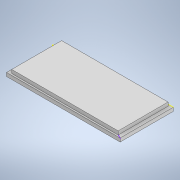
# Autodesk Inventor part: kansi
Saved by Autodesk Inventor 2020.1 (Build 241239000, 239)
## iProperties
Created: 2021-11-03
Part Number: kansi
Material: Generic
Document SubType Name: Modeling
Designer: s1mate03
Density: 1 g/cm^3
Appearance: Default
Author: s1mate03
Autodesk Inventor part; units mm, degrees
ref_plane "YZ Plane" through (0, 0, 0) normal (1, 0, 0) x (0, 1, 0)
ref_plane "XZ Plane" through (0, 0, 0) normal (0, 1, 0) x (-1, 0, 0)
ref_plane "XY Plane" through (0, 0, 0) normal (0, 0, 1) x (1, 0, 0)
sketch "Sketch1" plane through (0, 0, 0) normal (0, 1, 0) x (-1, 0, 0)
  line L0 (0, 13.1214) -> (-32, 13.1214)
  line L1 (-32, 13.1214) -> (-32, -1.8786)
  line L2 (-32, -1.8786) -> (0, -1.8786)
  line L3 (0, -1.8786) -> (0, 13.1214)
  point P0 (0, 0)
  dimension "d0" = 32
  dimension "d1" = 15
  constraints: 8 end point, 2 parallel, 1 horizontal, 1 perpendicular
  measures "d0" distance of L2.end L1.end
  measures "d1" distance of L1.end L0.end
extrude "Extrusion1" add sketch "Sketch1" along normal blind 1
sketch "Sketch2" plane through (0, 1, 0) normal (0, 1, 0) x (1, 0, 0)
  line L0 (32, 1.8786) -> (0, 1.8786) projected
  line L1 (32.1041, -13.1869) -> (0, 1.8786)
  point P0 (0, 0)
  constraints: 2 end point
sketch "Sketch3" plane through (0, 1, 0) normal (0, 1, 0) x (1, 0, 0)
  line L0 (31.001, -12.6665) -> (0.9997, -12.6665)
  line L1 (0.9997, -12.6665) -> (0.9997, 1.4049)
  line L2 (0.9997, 1.4049) -> (31.001, 1.4049)
  line L3 (31.001, 1.4049) -> (31.001, -12.6665)
  point P0 (0, 0)
  constraints: 8 end point, 2 parallel, 1 horizontal, 1 perpendicular
extrude "Extrusion2" add sketch "Sketch3" along normal blind 1
body "Solid1"
